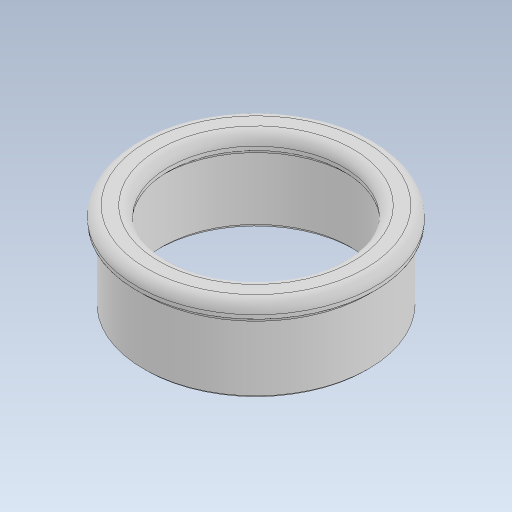
# Autodesk Inventor part: mesh-reseater
Saved by Autodesk Inventor 2023 (Build 270158030, 158C)
## iProperties
Created: 2024-10-09
Part Number: mesh-reseater
Material: Generic
Document SubType Name: Modeling
Designer: Imogen Heard
Density: 1 g/cm^3
Appearance: Default
Author: Imogen Heard
Autodesk Inventor part; units mm, degrees
ref_plane "YZ Plane" through (0, 0, 0) normal (1, 0, 0) x (0, 1, 0)
ref_plane "XZ Plane" through (0, 0, 0) normal (0, 1, 0) x (-1, 0, 0)
ref_plane "XY Plane" through (0, 0, 0) normal (0, 0, 1) x (1, 0, 0)
sketch "Sketch1" plane through (0, 0, 0) normal (0, 1, 0) x (-1, 0, 0)
  circle A0 centre (0, 0) radius 23
  circle A1 centre (0, 0) radius 19.25
  dimension "d2" = 46
  dimension "d3" = 38.5
  constraints: 2 centre point, 1 coincident
  measures "d2" diameter of A0
  measures "d3" diameter of A1
extrude "Extrusion1" add sketch "Sketch1" along normal blind 18 draft 5
sketch "Sketch2" plane through (0, 0, 0) normal (0, -1, 0) x (1, 0, 0)
  circle A0 centre (0, 0) radius 19.25 projected
  circle A1 centre (0, 0) radius 23 projected
  circle A2 centre (0, 0) radius 24.5748 projected
  circle A3 centre (0, 0) radius 17.6752 projected
extrude "Extrusion2" cut sketch "Sketch2" against normal blind 15 contours A0 | A2 | A3
chamfer "Chamfer1" distance 1.3 angle 45 1 edges at (-23, 15, 0)
chamfer "Chamfer2" distance 1 angle 45 1 edges at (-19.25, 0, 0)
chamfer "Chamfer3" distance 0.5 angle 45 1 edges at (-23, 0, 0)
fillet "Fillet1" radius 2 2 edges at (17.6752, 18, 0) (24.5748, 18, 0)
chamfer "Chamfer4" distance 1.3 angle 45 1 edges at (-19.25, 15, 0)
body "Solid1"
